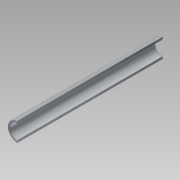
# Autodesk Inventor part: tube
Saved by Autodesk Inventor 2014 (Build 180170000, 170)
## iProperties
Created: 2013-10-04
Part Number: tube
Material: Glass
Document SubType Name: Modeling
Designer: Admin
Density: 1 g/cm^3
Appearance: Clear
Author: Admin
Autodesk Inventor part; units mm, degrees
ref_plane "YZ Plane" through (0, 0, 0) normal (1, 0, 0) x (0, 1, 0)
ref_plane "XZ Plane" through (0, 0, 0) normal (0, 1, 0) x (-1, 0, 0)
ref_plane "XY Plane" through (0, 0, 0) normal (0, 0, 1) x (1, 0, 0)
sketch "Sketch3" plane through (0, 0, 0) normal (0, 1, 0) x (-1, 0, 0)
  circle A0 centre (0, 0) radius 4
  circle A1 centre (0, 0) radius 3
  dimension "d4" = 8
  dimension "d6" = 6
  constraints: 2 centre point, 2 coincident
  measures "d4" diameter of A0
  measures "d6" diameter of A1
extrude "Extrusion2" add sketch "Sketch3" along normal blind 60
fillet "Fillet1" radius 0.3 2 edges at (4, 0, 0) (3, 0, 0)
fillet "Fillet2" radius 0.3 1 edges at (4, 60, 0)
fillet "Fillet3" radius 0.3 1 edges at (3, 60, 0)
body "Solid2"
